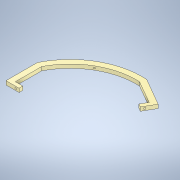
# Autodesk Inventor part: insert_8in
Saved by Autodesk Inventor 2021 (Build 250183000, 183)
## iProperties
Created: 2020-10-07
Part Number: insert_8in
Material: Generic
Document SubType Name: Modeling
Designer: dsouthall
Density: 1 g/cm^3
Appearance: Default
Author: dsouthall
Autodesk Inventor part; units mm, degrees
ref_plane "YZ Plane" through (0, 0, 0) normal (1, 0, 0) x (0, 1, 0)
ref_plane "XZ Plane" through (0, 0, 0) normal (0, 1, 0) x (-1, 0, 0)
ref_plane "XY Plane" through (0, 0, 0) normal (0, 0, 1) x (1, 0, 0)
sketch "Sketch1" plane through (0, 0, 0) normal (0, 1, 0) x (-1, 0, 0)
  line L0 (226.205, -0.8) -> (-105.3043, -0.8) construction
  line L1 (226.205, 0) -> (0, 0) construction
  line L2 (0, 0) -> (-124.0509, -214.8625) construction
  line L3 (-123.3581, -215.2625) -> (29.3027, 49.1538) construction
  line L4 (226.205, -5.88) -> (-105.3043, -5.88) construction
  line L5 (-118.9587, -217.8025) -> (33.7021, 46.6138) construction
  line L6 (70.231, -0.8) -> (88.011, -0.8)
  line L7 (88.011, -0.8) -> (88.011, -43.4926)
  line L8 (80.391, -5.88) -> (80.391, -41.6746)
  line L9 (70.231, -0.8) -> (70.231, -5.88)
  line L10 (70.231, -5.88) -> (80.391, -5.88)
  line L11 (-43.3127, -76.6198) -> (-6.3398, -97.9661)
  line L12 (-35.1033, -72.5606) -> (-4.1043, -90.4579)
  arc A0 (-4.1043, -90.4579) -> (80.391, -41.6746) centre (0, 0) ccw
  arc A1 (-6.3398, -97.9661) -> (88.011, -43.4926) centre (0, 0) ccw
  line L13 (-43.3127, -76.6198) -> (-34.4227, -61.2218)
  line L14 (-34.4227, -61.2218) -> (-30.0233, -63.7618)
  line L15 (-30.0233, -63.7618) -> (-35.1033, -72.5606)
  arc A2 (88.011, -43.4926) -> (98.171, 0) centre (0, 0) ccw construction
  line L16 (74.671, -0.8) -> (74.671, -5.88) construction
  line L17 (0, 0) -> (66.0288, -114.3653) construction
  dimension "d5" = 0.8
  dimension "d6" = 0.8
  dimension "d7" = 120
  dimension "d8" = 5.08
  dimension "d9" = 5.08
  dimension "d13" = 90
  dimension "d14" = 88.011
  dimension "d15" = 7.62
  dimension "d16" = 70.231
  dimension "d17" = 90
  dimension "d19" = 7.62
  dimension "d20" = 70.231
  dimension "d21" = 17.78
  dimension "d22" = 98.171
  dimension "d23" = 90.551
  dimension "d24" = 23.5
  dimension "d46" = 60
  constraints: 36 end point, 11 point on line, 6 point on circle, 5 parallel, 3 centre point, 3 coincident, 2 horizontal, 2 perpendicular, 1 collinear, 1 vertical
  measures "d5" distance between parallel lines of L1 L0
  measures "d6" distance between parallel lines of L2 L3
  measures "d7" angle of L2 L1
  measures "d8" distance between parallel lines of L0 L4
  measures "d9" distance between parallel lines of L3 L5
  measures "d13" angle of L0 L7
  measures "d14" horizontal distance of point (0, 0) L6.end
  measures "d15" distance between parallel lines of L7 L8
  measures "d16" horizontal distance of point (0, 0) L6.start
  measures "d17" angle of L3 L11
  measures "d19" distance between parallel lines of L12 L11
  measures "d20" distance from line of point (0, 0) L14
  measures "d21" distance of L11.start L13.end
  measures "d22" radius of A1
  measures "d23" radius of A0
  measures "d24" horizontal distance of L16.start A2.end
  measures "d46" angle of L17 L1
extrude "Extrusion1" add sketch "Sketch1" along normal blind 5.08
ref_plane "radial plane for hole1" through (0, 0, 0) normal (0, 0, 1) x (1, 0, 0)
sketch "sketch hole 1" plane through (0, 0, 0) normal (0, 0, 1) x (1, 0, 0)
  line L0 (-74.671, 0) -> (-74.671, 5.08) construction
  line L1 (-88.011, 5.08) -> (-70.231, 5.08) projected
  point P0 (0, 0)
  point P1 (-74.671, 2.54)
  dimension "d28" = 74.671
  dimension "d29" = 2.54
  constraints: 2 end point, 1 midpoint, 1 vertical
  measures "d28" distance from line of point (0, 0) L0
  measures "d29" distance from line of L1 point (-74.671, 2.54)
ref_plane "radial plane for hole2" through (0, 0, 0) normal (0.8660254, 0, 0.5) x (0.5, 0, -0.8660254)
hole "Hole2" at (37.3355, 2.54, -64.667) direction (-0.8660254, 0, -0.5) diameter 2.4384 depth 12.2936 tip angle 118 clearance for "Flat Head Machine Screw (82)" size "#2" standard "Ansi Unified Screw Threads"
sketch "sketch hole 2" plane through (0, 0, 0) normal (0.8660254, 0, 0.5) x (0.5, 0, -0.8660254)
  line L0 (74.671, 5.3744) -> (74.671, -0.2944) construction
  line L1 (70.231, 5.08) -> (88.011, 5.08) construction
  point P0 (0, 0)
  point P1 (74.671, 2.54)
  dimension "d30" = 74.671
  dimension "d31" = 2.54
  constraints: 2 end point, 1 midpoint, 1 vertical
  measures "d30" distance from line of point (0, 0) L0
  measures "d31" distance from line of L1 point (74.671, 2.54)
hole "Hole1" at (-74.671, 2.54, 0) direction (0, 0, -1) diameter 2.4384 depth 12.2936 tip angle 118 clearance for "Flat Head Machine Screw (82)" size "#2" standard "Ansi Unified Screw Threads"
ref_plane "tangential plane for hole3" through (-49.0855, 0, -85.0186) normal (-0.5, 0, -0.8660254) x (0, -1, 0)
sketch "Sketch6" plane through (-49.0855, 0, -85.0186) normal (-0.5, 0, -0.8660254) x (0, -1, 0)
  point P0 (0, 0)
  point P1 (-2.54, 0)
  dimension "d47" = 2.54
  dimension "d48" = 0
  measures "d47" distance of point (-2.54, 0) point (0, 0)
  measures "d48" vertical distance of point (0, 0) point (-2.54, 0)
hole "Hole3" at (-49.0855, 2.54, -85.0186) direction (0.5, 0, 0.8660254) diameter 2.1565 depth 8.8646 tip angle 118 thread size "4-40 UNC" class "2B" standard "ANSI Unified Screw Threads"
equation "\"d6\" = d5"
equation "\"d9\" = d8"
equation "\"d17\" = d13"
equation "\"d19\" = d15"
equation "\"d20\" = d16"
equation "\"d21\" = d14 - d16"
equation "\"d46\" = 0.5 * d7"
equation "\"d28\" = d22 - d24"
equation "\"d30\" = d28"
body "Solid1"
